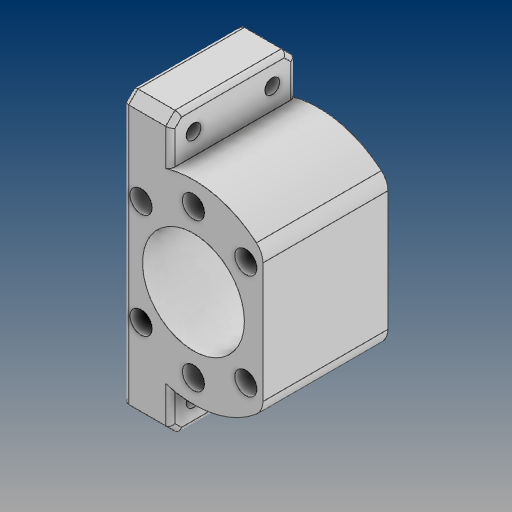
# Autodesk Inventor part: 18_Khoi_vuong_1204
Saved by Autodesk Inventor 2021 (Build 250183000, 183)
## iProperties
Created: 2024-04-06
Part Number: 18_Khoi_vuong_1204
Material: Generic
Document SubType Name: Modeling
Designer: Admin
Density: 1 g/cm^3
Appearance: Default
Author: Admin
Autodesk Inventor part; units mm, degrees
ref_plane "YZ Plane" through (0, 0, 0) normal (1, 0, 0) x (0, 1, 0)
ref_plane "XZ Plane" through (0, 0, 0) normal (0, 1, 0) x (-1, 0, 0)
sketch "Sketch1" plane through (0, 0, 0) normal (0, 0, 1) x (1, 0, 0)
  line L0 (-15, 30) -> (15, 30)
  line L1 (15, 30) -> (15, -30)
  line L2 (15, -30) -> (-15, -30)
  line L3 (-15, -30) -> (-15, 30)
  line L4 (-15, 30) -> (15, -30) construction
  line L5 (15, 30) -> (-15, -30) construction
  circle A0 centre (11.3137, -11.3137) radius 2.4 projected
  circle A1 centre (0, -16) radius 2.4 projected
  circle A2 centre (-11.3137, -11.3137) radius 2.4 projected
  circle A3 centre (-11.3137, 11.3137) radius 2.4 projected
  circle A4 centre (11.3137, 11.3137) radius 2.4 projected
  circle A5 centre (0, 16) radius 2.4 projected
  line L6 (-15, 14.6969) -> (-15, -14.6969) projected
  arc A6 (-15, -14.6969) -> (15, -14.6969) centre (0, 0) ccw projected
  line L7 (15, -14.6969) -> (15, 14.6969) projected
  arc A7 (15, 14.6969) -> (-15, 14.6969) centre (0, 0) ccw projected
  circle A8 centre (0, 0) radius 11 projected
  dimension "d0" = 30
  dimension "d1" = 60
  dimension "d2" = 30
  dimension "d3" = 21
  constraints: 12 end point, 2 midpoint, 2 parallel, 1 horizontal, 1 perpendicular
  measures "d0" distance between parallel lines of L3 L1
  measures "d1" distance between parallel lines of L0 L2
  measures "d2" distance between parallel lines of L6 L7
  measures "d3" radius of A7
ref_plane "Work Plane1" through (-10.75, -10.75, 27) normal (0, 0, 1) x (1, 0, 0)
extrude "Extrusion1" add sketch "Sketch1" along normal up to surface (27 mm away)
sketch "Sketch2" plane through (15, -30, 0) normal (1, 0, 0) x (0, 0, -1)
  line L0 (-27, 16.4) -> (-27, 11.6) projected
  line L1 (0, 11.6) -> (0, 16.4) projected
  line L2 (-27, 48.4) -> (-27, 43.6) projected
  line L3 (0, 43.6) -> (0, 48.4) projected
  line L4 (0, 43.6) -> (0, 48.4) projected
  line L5 (0, 46) -> (-27, 46) construction
  line L6 (-27, 48.4) -> (-27, 43.6) projected
  line L7 (0, 11.6) -> (0, 16.4) projected
  line L8 (0, 14) -> (-27, 14) construction
  line L9 (0, 5) -> (-27, 5)
  line L10 (-27, 60) -> (-27, 0) projected
  line L11 (0, 0) -> (-27, 0) projected
  line L12 (0, 30) -> (-27, 30) construction
  line L13 (0, 55) -> (-27, 55)
  line L14 (0, 60) -> (-27, 60) projected
  line L15 (-13.5, 60) -> (-13.5, 0) construction
  line L16 (0, 0) -> (0, 60) projected
  point P0 (-5, 55)
  point P1 (-5, 5)
  point P2 (-22, 55)
  point P3 (-22, 5)
  dimension "d7" = 5
  dimension "d9" = 5
  constraints: 12 end point, 6 midpoint, 5 symmetric about line, 4 point on line, 2 horizontal, 1 perpendicular, 3 other
  measures "d7" distance between parallel lines of L11 L9
hole "Hole1" at (15, 25, 5) at (15, -25, 5) at (15, 25, 22) at (15, -25, 22) direction (-1, 0, 0) diameter 3.2 end through all
sketch "Sketch3" plane through (-15, 30, 27) normal (0, 0, 1) x (1, 0, 0)
  circle A0 centre (15, -30) radius 6 projected
  circle A1 centre (26.3137, -41.3137) radius 2.4 projected
  circle A2 centre (15, -46) radius 2.4 projected
  circle A3 centre (3.6863, -41.3137) radius 2.4 projected
  circle A4 centre (3.6863, -18.6863) radius 2.4 projected
  circle A5 centre (26.3137, -18.6863) radius 2.4 projected
  circle A6 centre (15, -14) radius 2.4 projected
  line L0 (0, -44.6969) -> (0, -15.3031) projected
  arc A7 (30, -15.3031) -> (0, -15.3031) centre (15, -30) ccw projected
  line L1 (30, -15.3031) -> (30, -44.6969) projected
  arc A8 (0, -44.6969) -> (30, -44.6969) centre (15, -30) ccw projected
  line L2 (0, -56.6) -> (30, -56.6) projected
  circle A9 centre (15, -30) radius 11 projected
  circle A10 centre (15, -14) radius 2.4 projected
  circle A11 centre (26.3137, -18.6863) radius 2.4 projected
  circle A12 centre (3.6863, -18.6863) radius 2.4 projected
  circle A13 centre (3.6863, -41.3137) radius 2.4 projected
  circle A14 centre (15, -46) radius 2.4 projected
  circle A15 centre (26.3137, -41.3137) radius 2.4 projected
  line L3 (0, 0) -> (30, 0) projected
  line L4 (0, -60) -> (0, 0) projected
  line L5 (30, -60) -> (0, -60) projected
  line L6 (30, 0) -> (30, -60) projected
  line L7 (10, -9.6039) -> (10, 0)
  line L8 (30, 0) -> (0, 0) projected
  line L9 (10, -50.3961) -> (10, -60)
  point P0 (30, -15.3031)
  dimension "d17" = 10
  constraints: 4 end point, 4 point on line, 2 point on circle, 1 vertical
  measures "d17" distance between parallel lines of L4 L7
extrude "Extrusion2" cut sketch "Sketch3" against normal through all contours A8 L6 L2 L9 | L7 L3 L6 A7 | L2 L6 L5 L9
chamfer "Chamfer1" distance 2 angle 45 4 edges at (-10, 30, 27) (-10, 30, 0) (-10, -30, 0) (-10, -30, 27)
fillet "Fillet1" radius 4 2 edges at (15, -14.6969, 13.5) (15, 14.6969, 13.5)
fillet "Fillet2" radius 1 10 edges at (-5, 29, 1) (-5, 30, 13.5) (-5, 29, 26) (-5, 24.198, 27) (-5, 24.198, 0) (-5, -29, 26) (-5, -30, 13.5) (-5, -29, 1) (-5, -24.198, 0) (-5, -24.198, 27)
fillet "Fillet3" radius 1 8 edges at (-15, -29, 26) (-15, 0, 27) (-15, 29, 26) (-15, 30, 13.5) (-15, 29, 1) (-15, 0, 0) (-15, -29, 1) (-15, -30, 13.5)
equation "\"d0\" = d2"
body "Solid1"
